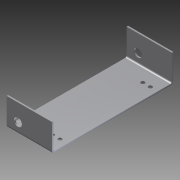
# Autodesk Inventor part: MotorPlatta
Saved by Autodesk Inventor 2014 (Build 180170000, 170)
## iProperties
Created: 2014-02-18
Part Number: MotorPlatta
Material: Generic
Document SubType Name: Sheet Metal
Designer: Pinkponk
Density: 1 g/cm^3
Sheet Metal Rule: Default_mm
Flat Pattern Width: 6 cm
Flat Pattern Length: 22.8048 cm
Flat Pattern Area: 136.829 cm^2
Sheet Metal Width: 60,000 mm
Sheet Metal Length: 228,048 mm
Sheet Metal Area: 13682,867 mm^2
Appearance: Default
Author: Pinkponk
Autodesk Inventor part; units mm, degrees
ref_plane "YZ Plane" through (0, 0, 0) normal (1, 0, 0) x (0, 1, 0)
ref_plane "XZ Plane" through (0, 0, 0) normal (0, 1, 0) x (-1, 0, 0)
ref_plane "XY Plane" through (0, 0, 0) normal (0, 0, 1) x (1, 0, 0)
sketch "Sketch1" plane through (0, 0, 0) normal (0, 0, 1) x (1, 0, 0)
  line L0 (0, 0) -> (60, 0)
  line L1 (60, 0) -> (60, 153)
  line L2 (60, 153) -> (0, 153)
  line L3 (0, 153) -> (0, 0)
  dimension "d0" = 153
  dimension "d1" = 60
  measures "d0" distance of L2.end L0.start
  measures "d1" distance of L1.end L2.end
extrude "Plate1" add sketch "Sketch1" along normal blind 2
sketch "Sketch2" plane through (60, -2, 4) normal (0, -1, 0) x (1, 0, 0)
  line L0 (-60, 0) -> (0, 0)
  line L1 (0, 0) -> (0, 33)
  line L2 (0, 33) -> (-60, 33)
  line L3 (-60, 33) -> (-60, 0)
  constraints: 6 end point, 1 horizontal, 1 perpendicular, 1 vertical
edge flange "Flange1" height 35 angle 90 thickness 2 bend radius 2 thickness toward (0, -1, 0) relief tear relief width 2 relief depth 1 corner gap 2 corner form 0 edges at (30, 0, 2) (30, 153, 2) wall of the first edge with corners at (0, -2, 4) (60, -2, 4) (60, -2, 37) (0, -2, 37)
bend "Bend1"
corner "Corner1"
sketch "Sketch3" plane through (0, -4, 37) normal (0, -1, 0) x (1, 0, 0)
  line L0 (0, -33) -> (60, -33) projected
  line L1 (0, -33) -> (0, 0) projected
  circle A0 centre (15, -22.75) radius 5.25
  point P0 (0, -37)
  dimension "d13" = 15
  dimension "d14" = 10.5
  dimension "d16" = 10.25
  constraints: 1 centre point
  measures "d13" distance from line of L1 A0.centre
  measures "d14" diameter of A0
  measures "d16" distance from line of L0 A0.centre
extrude "Extrusion1" cut sketch "Sketch3" against normal through all
sketch "Sketch4" plane through (0, 0, 2) normal (0, 0, 1) x (1, 0, 0)
  line L0 (0, 0) -> (0, 153) projected
  line L1 (60, 153) -> (60, 0) projected
  circle A0 centre (50, 136.5) radius 2.5
  circle A1 centre (40, 136.5) radius 2.5
  line L2 (60, 76.5) -> (0, 76.5) construction
  circle A2 centre (50, 16.5) radius 2.5
  circle A3 centre (40, 16.5) radius 2.5
  dimension "d20" = 10
  dimension "d21" = 20
  dimension "d22" = 5
  dimension "d23" = 5
  dimension "d24" = 120
  constraints: 4 centre point, 2 end point, 2 midpoint, 2 symmetric about line, 1 horizontal alignment, 2 other
  measures "d20" distance from line of A0.centre L1
  measures "d21" distance from line of L1 A1.centre
  measures "d22" diameter of A1
  measures "d23" diameter of A0
  measures "d24" distance of A2.centre A0.centre
extrude "Extrusion2" cut sketch "Sketch4" against normal through all
equation "\"d3\" = BendReliefWidth"
equation "\"d4\" = BendReliefDepth"
equation "\"d5\" = MinimumRemnant"
equation "\"d6\" = BendRadius"
equation "\"d9\" = BendRadius"
equation "\"d10\" = CornerReliefSize"
equation "\"d11\" = GapSize"
equation "\"d12\" = JacobiRadiusSize"
equation "\"BendRadius\" = Thickness"
equation "\"BendReliefWidth\" = Thickness"
equation "\"BendReliefDepth\" = 0.5 * Thickness"
equation "\"CornerReliefSize\" = 4 * Thickness"
equation "\"MinimumRemnant\" = 2 * Thickness"
equation "\"TransitionRadius\" = BendRadius"
equation "\"JacobiRadiusSize\" = BendRadius"
equation "\"GapSize\" = Thickness"
equation "\"d2\" = BendRadius"
equation "\"Thickness\" = 2"
body "Solid1"
